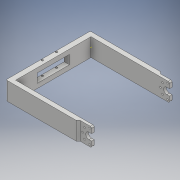
# Autodesk Inventor part: shoulder_gear_3
Saved by Autodesk Inventor 2018 (Build 220112000, 112)
## iProperties
Created: 2020-09-07
Part Number: shoulder_gear_3
Material: 일반
Document SubType Name: Modeling
Designer: j3jjj
Density: 1 g/cm^3
Appearance: 기본값
Author: j3jjj
Autodesk Inventor part; units mm, degrees
ref_plane "YZ Plane" through (0, 0, 0) normal (1, 0, 0) x (0, 1, 0)
ref_plane "XZ Plane" through (0, 0, 0) normal (0, 1, 0) x (-1, 0, 0)
ref_plane "XY Plane" through (0, 0, 0) normal (0, 0, 1) x (1, 0, 0)
sketch "스케치1" plane through (0, 0, 0) normal (0, 1, 0) x (-1, 0, 0)
  line L0 (65, -14) -> (-65, -14)
  line L1 (-65, -14) -> (-65, 14)
  line L2 (-65, 14) -> (65, 14)
  line L3 (65, 14) -> (65, -14)
  point P0 (0, 0)
  dimension "d0" = 28
  dimension "d1" = 130
  dimension "d2" = 14
  dimension "d3" = 65
  constraints: 8 end point, 2 parallel, 1 horizontal, 1 perpendicular
  measures "d0" distance between parallel lines of L0 L2
  measures "d1" distance between parallel lines of L1 L3
  measures "d2" distance from line of L2 point (0, 0)
  measures "d3" distance from line of point (0, 0) L3
extrude "돌출1" add sketch "스케치1" along normal blind 7
sketch "스케치4" plane through (0, 0, 0) normal (0, -1, 0) x (1, 0, 0)
  line L0 (-65, -14) -> (65, -14) projected
  line L1 (65, 14) -> (-65, 14) projected
  line L2 (-65, -14) -> (-57, -14)
  line L3 (-57, -14) -> (-57, 14)
  line L4 (-57, 14) -> (-65, 14)
  line L5 (-65, 14) -> (-65, -14)
  point P0 (0, 0)
  point P1 (63, -14)
  point P2 (63, 14)
  dimension "d26" = 8
  constraints: 8 end point, 2 parallel, 1 horizontal, 1 perpendicular, 1 point on line
  measures "d26" distance between parallel lines of L5 L3
extrude "돌출4" add sketch "스케치4" along normal blind 124
fillet "모깎기2" radius 2 1 edges at (-65, 7, 0)
sketch "스케치5" plane through (-57, 0, 14) normal (1, 0, 0) x (0, 0, -1)
  point P0 (14, 0)
sketch "스케치10" plane through (-57, 0, 14) normal (1, 0, 0) x (0, 0, -1)
  line L0 (0, -124) -> (28, -124) projected
  line L1 (28, -124) -> (28, 5) projected
  line L2 (0, -124) -> (28, -124)
  line L3 (28, -124) -> (28, -117)
  line L4 (28, -117) -> (0, -117)
  line L5 (0, -117) -> (0, -124)
  point P0 (14, 0)
  dimension "d52" = 7
  constraints: 8 end point, 2 parallel, 1 horizontal, 1 perpendicular, 1 point on line
  measures "d52" distance between parallel lines of L4 L0
extrude "돌출9" add sketch "스케치10" along normal blind 122
sketch "스케치2" plane through (0, 7, 0) normal (0, 1, 0) x (1, 0, 0)
  circle A0 centre (61, 0) radius 5
  line L0 (61, 5) -> (65, 5)
  line L1 (65, 5) -> (65, -5)
  line L2 (65, -5) -> (61, -5)
  line L3 (61, -5) -> (61, 5)
  line L4 (65, -14) -> (65, 14) projected
  point P0 (0, 0)
  dimension "d6" = 10
  dimension "d7" = 0
  dimension "d8" = 10
  dimension "d9" = 5
  dimension "d10" = 4
  dimension "d11" = 0
  constraints: 8 end point, 2 parallel, 1 centre point, 1 horizontal, 1 perpendicular
  measures "d6" diameter of A0
  measures "d7" distance between parallel lines of L1 L4
  measures "d8" distance between parallel lines of L0 L2
  measures "d9" distance from line of point (0, 0) L2
  measures "d10" distance between parallel lines of L1 L3
  measures "d11" distance from line of A0.centre L3
extrude "돌출2" cut sketch "스케치2" against normal blind 180
sketch "스케치3" plane through (0, 7, 0) normal (0, 1, 0) x (1, 0, 0)
  circle A0 centre (62, 11) radius 1.25
  line L0 (65, 5) -> (65, 14) projected
  line L1 (65, 14) -> (-65, 14) projected
  line L2 (0, 0) -> (4.9885, 0)
  circle A1 centre (62, -11) radius 1.25
  circle A2 centre (51, 0) radius 1.25
  line L3 (-65, -14) -> (65, -14) projected
  circle A3 centre (54.222, -7.778) radius 1.25
  line L4 (65, -14) -> (65, -5) projected
  circle A4 centre (54.222, 7.778) radius 1.25
  dimension "d14" = 2.5
  dimension "d15" = 3
  dimension "d16" = 3
  dimension "d17" = 14
  dimension "d18" = 2.5
  dimension "d19" = 14
  dimension "d20" = 10.778
  dimension "d21" = 6.222
  dimension "d22" = 2.5
  constraints: 5 centre point, 2 end point, 2 symmetric about line, 1 horizontal, 2 other
  measures "d14" diameter of A0
  measures "d15" distance from line of L0 A0.centre
  measures "d16" distance from line of L1 A0.centre
  measures "d17" distance from line of L0 A2.centre
  measures "d18" diameter of A2
  measures "d19" distance from line of L3 A2.centre
  measures "d20" distance from line of L4 A3.centre
  measures "d21" distance from line of L3 A3.centre
  measures "d22" diameter of A3
extrude "돌출3" cut sketch "스케치3" against normal blind 100000
fillet "모깎기4" radius 2 5 edges at (65, -120.5, 14) (65, -120.5, -14) (65, 3.5, -14) (65, 3.5, 14) (-65, -124, 0)
sketch "스케치11" plane through (-57, -117, 14) normal (0, 0, 1) x (1, 0, 0)
  circle A0 centre (-6, 47.5) radius 1.5
  circle A1 centre (-6, 69.5) radius 1.5
  line L0 (-8, 122) -> (-8, -5) projected
  line L1 (181.1056, 58.5) -> (-67.096, 58.5)
  point P0 (57, 117)
  dimension "d56" = 3
  dimension "d57" = 3
  dimension "d58" = 2
  dimension "d59" = 2
  dimension "d60" = 22
  dimension "d61" = 58.5
  dimension "d62" = 11
  constraints: 2 centre point, 2 end point, 1 horizontal
  measures "d56" diameter of A0
  measures "d57" diameter of A1
  measures "d58" distance from line of L0 A0.centre
  measures "d59" distance from line of L0 A1.centre
  measures "d60" distance of A1.centre A0.centre
  measures "d61" distance from line of point (57, 117) L1
  measures "d62" distance from line of L1 A0.centre
extrude "돌출10" cut sketch "스케치11" against normal blind 122
sketch "스케치12" plane through (-57, 0, 14) normal (1, 0, 0) x (0, 0, -1)
  line L0 (7, -33.5) -> (21, -33.5)
  line L1 (21, -33.5) -> (21, -83.5)
  line L2 (21, -83.5) -> (7, -83.5)
  line L3 (7, -83.5) -> (7, -33.5)
  line L4 (0, 0) -> (0, -117) projected
  line L5 (28, 0) -> (28, -117) projected
  line L6 (-36.3144, -58.5) -> (56.0369, -58.5)
  line L7 (9, -117) -> (19, -117) projected
  point P0 (14, 0)
  dimension "d65" = 7
  dimension "d66" = 7
  dimension "d67" = 50
  dimension "d68" = 58.5
  dimension "d69" = 25
  constraints: 10 end point, 2 horizontal, 2 parallel, 1 perpendicular
  measures "d65" distance between parallel lines of L3 L4
  measures "d66" distance between parallel lines of L5 L1
  measures "d67" distance between parallel lines of L0 L2
  measures "d68" distance between parallel lines of L6 L7
  measures "d69" distance between parallel lines of L6 L2
extrude "돌출11" cut sketch "스케치12" against normal blind 122
sketch "스케치13" plane through (0, -124, 0) normal (0, -1, 0) x (1, 0, 0)
  line L0 (-63, 14) -> (63, 14) projected
  line L1 (47, 14) -> (65, 14)
  line L2 (65, 14) -> (65, -15.4156)
  line L3 (65, -15.4156) -> (47, -15.4156)
  line L4 (47, -15.4156) -> (47, 14)
  line L5 (65, 12) -> (65, 5) projected
  point P0 (0, 0)
  dimension "d72" = 18
  dimension "d73" = 0
  constraints: 8 end point, 2 parallel, 1 horizontal, 1 perpendicular, 1 point on line
  measures "d72" distance between parallel lines of L2 L4
  measures "d73" distance between parallel lines of L5 L2
extrude "돌출12" cut sketch "스케치13" against normal blind 3
sketch "스케치14" plane through (0, 7, 0) normal (0, 1, 0) x (1, 0, 0)
  line L0 (-57, -14) -> (63, -14) projected
  line L1 (-57, 14) -> (63, 14) projected
  line L2 (47, -14) -> (65, -14)
  line L3 (65, -14) -> (65, 14)
  line L4 (65, 14) -> (47, 14)
  line L5 (47, 14) -> (47, -14)
  line L6 (65, -12) -> (65, -5) projected
  point P0 (0, 0)
  dimension "d76" = 18
  dimension "d77" = 0
  constraints: 8 end point, 2 parallel, 2 point on line, 1 horizontal, 1 perpendicular
  measures "d76" distance between parallel lines of L3 L5
  measures "d77" distance between parallel lines of L6 L3
extrude "돌출13" cut sketch "스케치14" against normal blind 3
chamfer "모따기1" distance 3 angle 45 2 edges at (47, 7, 0) (47, -124, 0)
